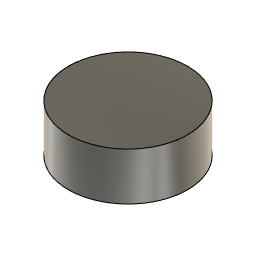
speed_meter (Autodesk Fusion 360 archive; units mm, degrees)
design "magnes"
Autodesk Fusion 360 part; units mm, degrees
note: some values were not read from the file. Chosen so that the rebuilt part matches the saved one: a direction; which face or edge a step refers to. Set by a fixed rule: which sketch regions a step uses.
sketch "Szkic1" plane through (0, 0, 0) normal (0, 0, 1) x (1, 0, 0)
  circle A0 centre (0, 0) radius 5
  dimension "d1" = 10
  constraint coincident A0.centre origin
  measures "d1" diameter of A0
extrude "Wyciągnięcie proste1" add sketch "Szkic1" along normal blind 4

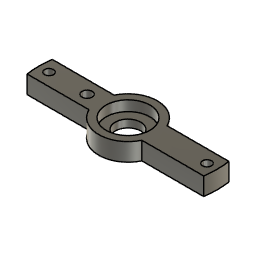
design "podstawa"
Autodesk Fusion 360 part; units mm, degrees
sketch "Szkic1" plane through (0, 0, 0) normal (0, 0, 1) x (1, 0, 0)
  circle A0 centre (0, 0) radius 11.5
  circle A1 centre (0, 0) radius 8.6
  circle A2 centre (0, 0) radius 5
  dimension "d1" = 23
  dimension "d2" = 17.2
  dimension "d7" = 10
  constraint coincident A0.centre A1.centre
  measures "d1" diameter of A0
  measures "d2" diameter of A1
  measures "d7" diameter of A2
extrude "Wyciągnięcie proste1" add sketch "Szkic1" along normal blind 7 contours A0
extrude "Wyciągnięcie proste2" add sketch "Szkic1" along normal blind 3 contours A1
sketch "Szkic2" plane through (0, 0, 0) normal (0, 0, 1) x (1, 0, 0)
  line L0 (20, -5) -> (-20, -5)
  line L1 (-20, 5) -> (20, 5)
  line L2 (20, -5) -> (-20, 5) construction
  line L3 (-20, -5) -> (20, 5) construction
  line L4 (35, -4.95) -> (-35, -4.95)
  line L5 (-35, -4.95) -> (-35, 4.95)
  line L6 (-35, 4.95) -> (35, 4.95)
  line L7 (35, 4.95) -> (35, -4.95)
  line L8 (35, -4.95) -> (-35, 4.95) construction
  line L9 (-20, -5) -> (-24, -5)
  line L10 (-24, 5) -> (-20, 5)
  circle A0 centre (0, 0) radius 11.5
  line L11 (-35, -4.95) -> (-11.3867, -1.6104) construction
  line L12 (0, 0) -> (35, 4.95) construction
  circle A1 centre (0, 0) radius 35
  circle A2 centre (-31, 0) radius 1.75
  circle A3 centre (31, 0) radius 1.75
  circle A4 centre (-15.9999, -0.05) radius 2
  dimension "d9" = 10
  dimension "d10" = 70
  dimension "d11" = 9.9
  dimension "d36" = 3.5
  dimension "d37" = 4
  dimension "d38" = 4
  dimension "d68" = 4
  dimension "d69" = 5
  dimension "d70" = 16
  constraint horizontal L0
  constraint parallel L0 L1
  constraint coincident L2 A0.centre
  constraint coincident L3 A0.centre
  constraint coincident A0.centre L12.start
  constraint horizontal L4
  constraint perpendicular L4 L5
  constraint parallel L4 L6
  constraint parallel L5 L7
  constraint coincident L8 A0.centre
  constraint coincident A0.centre L11
  constraint horizontal L9
  constraint horizontal L10
  constraint coincident A0 L11.end
  constraint collinear L11 L12
  constraint tangent L7 A1
  constraint horizontal A0.centre A3.centre
  constraint horizontal A0.centre A2.centre
  constraint equal A2 A3
  measures "d9" distance of L0.end L1.start
  measures "d10" distance of L5.end L6.end
  measures "d11" distance of L4.end L5.end
  measures "d36" diameter of A3
  measures "d37" distance of L7 A3.centre
  measures "d38" distance of L5 A2.centre
  measures "d68" diameter of A4
  measures "d69" distance of L6 A4.centre
  measures "d70" distance of A0.centre A4.centre
extrude "Wyciągnięcie proste3" add sketch "Szkic2" along normal blind 7 contours L4 L6 A0 A1 | L4 L6 A0 A1

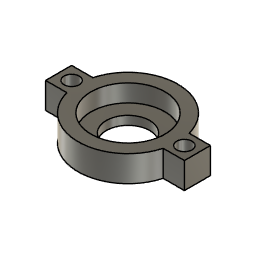
design "uchwyt lozysko"
Autodesk Fusion 360 part; units mm, degrees
sketch "Szkic1" plane through (0, 0, 0) normal (0, 0, 1) x (1, 0, 0)
  circle A0 centre (0, 0) radius 5
  circle A1 centre (0, 0) radius 8.5
  circle A2 centre (0, 0) radius 11.5
  circle A3 centre (13, 0) radius 1.75
  circle A4 centre (-13, 0) radius 1.75
  line L0 (16, 3) -> (-16, 3)
  line L1 (-16, 3) -> (-16, -3)
  line L2 (-16, -3) -> (16, -3)
  line L3 (16, -3) -> (16, 3)
  line L4 (16, 3) -> (-16, -3) construction
  line L5 (-16, 3) -> (16, -3) construction
  dimension "d1" = 10
  dimension "d2" = 17
  dimension "d3" = 23
  dimension "d4" = 3.5
  dimension "d5" = 13
  dimension "d6" = 3.5
  dimension "d7" = 13
  dimension "d8" = 32
  dimension "d9" = 6
  constraint coincident A0.centre A1.centre
  constraint concentric A0 A2
  constraint horizontal L0
  constraint perpendicular L0 L1
  constraint parallel L0 L2
  constraint parallel L1 L3
  constraint coincident L4 A0.centre
  constraint coincident L5 A0.centre
  constraint horizontal A0.centre A4.centre
  constraint horizontal A0.centre A3.centre
  measures "d1" diameter of A0
  measures "d2" diameter of A1
  measures "d3" diameter of A2
  measures "d4" diameter of A3
  measures "d5" distance of A0.centre A3.centre
  measures "d6" diameter of A4
  measures "d7" distance of A0.centre A4.centre
  measures "d8" distance of L1.end L2.end
  measures "d9" distance of L0.end L1.end
extrude "Wyciągnięcie proste1" add sketch "Szkic1" along normal blind 6 contours A1 A2 A3 L0 L2 | A1 A2 L0 | A1 A2 L2 | A1 A2 A4 L0 L2 | A2 A3 L0 L2 L3 | A2 A4 L0 L1 L2
extrude "Wyciągnięcie proste2" add sketch "Szkic1" along normal blind 2 contours A0 A1 L0 L2 | A0 A1 L0 | A0 A1 L2 | A0 A1 L0 L2

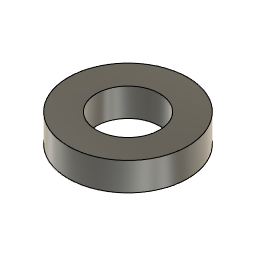
design "lozysko"
Autodesk Fusion 360 part; units mm, degrees
sketch "Szkic1" plane through (0, 0, 0) normal (0, 0, 1) x (1, 0, 0)
  circle A0 centre (0, 0) radius 4.5
  circle A1 centre (0, 0) radius 8.5
  dimension "d1" = 9
  dimension "d2" = 17
  constraint coincident A0.centre A1.centre
  constraint concentric A0 A1
  measures "d1" diameter of A0
  measures "d2" diameter of A1
extrude "Wyciągnięcie proste1" add sketch "Szkic1" along normal blind 4

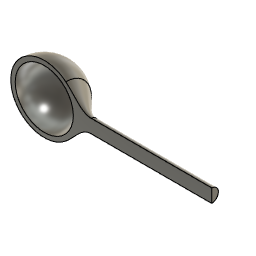
design "lopatka"
Autodesk Fusion 360 part; units mm, degrees
sketch "Szkic1" plane through (0, 0, 0) normal (0, 1, 0) x (1, 0, 0)
  line L0 (13, 0) -> (15, 0)
  line L1 (0, 0) -> (-15, 0)
  arc A0 (-15, 0) -> (15, 0) centre (0, 0) ccw
  arc A1 (-13, 0) -> (13, 0) centre (0, 0) ccw
  dimension "d1" = 30
  dimension "d2" = 26
  constraint coincident L1.start A0.centre
  constraint horizontal L0
  constraint parallel L0 L1
  constraint coincident L1 A1.start
  measures "d1" diameter of A0
  measures "d2" diameter of A1
revolve "Obrót1" add sketch "Szkic1" angle 180 about axis through (0, 0, 0) along (-1, 0, 0)
sketch "Szkic2" plane through (0, 0, 0) normal (0, 1, 0) x (1, 0, 0)
  line L0 (75, 0) -> (75, -3)
  line L1 (75, -3) -> (21, -3)
  spline S0 degree 5 poles (9.6157, -11.5125) (10.0753, -11.1286) (10.9799, -10.329) (12.293, -9.0341) (13.9792, -7.1799) (16.0934, -4.9797) (17.9027, -3.6587) (19.3902, -3.1198) (20.4518, -3) (21, -3) knots 0 0 0 0 0 0 0.2 0.4 0.6 0.8 1 1 1 1 1 1
  line L2 (8.6945, -12.2819) -> (10.5369, -10.7431)
  line L3 (20, -3) -> (22, -3)
  arc A0 (9.6157, -11.5125) -> (15, 0) centre (0, 0) ccw
  line L4 (15, 0) -> (75, 0)
  dimension "d9" = 60
  constraint vertical L0
  constraint horizontal L1
  constraint coincident A0.centre origin
  constraint midpoint S0.start L2
  constraint midpoint L1.end L3
  constraint coincident L1 L3.end
  constraint tangent L2 A0
  measures "d9" distance of A0.end L0.start
revolve "Obrót2" add sketch "Szkic2" angle 180 about axis through (1.75, 0, 0) along (-1, 0, 0) contours L0 L1 S0 L3 A0 L4

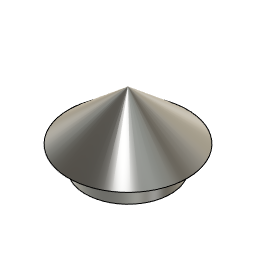
design "nakladka"
Autodesk Fusion 360 part; units mm, degrees
sketch "Szkic1" plane through (0, 0, 0) normal (0, 1, 0) x (1, 0, 0)
  line L0 (-6, 0) -> (0, -5.0346)
  line L1 (0, -3.3564) -> (0, -5.0346)
  line L2 (-2.5, 0) -> (1.3455, 0) construction
  line L3 (-2.5, 0) -> (0, -2.0977)
  line L4 (-2.5, 0) -> (1.1341, 0) construction
  line L5 (0, -2.0977) -> (0, -5.0346)
  line L6 (-2.5, 0) -> (-4, 1.2586)
  line L7 (-6, 0) -> (-4, 0) construction
  line L8 (-2.5, 0) -> (3.6054, 0) construction
  line L9 (-6, 0) -> (-8.0308, 1.704)
  line L10 (-8.0308, 1.704) -> (-6, 1.704)
  line L11 (-6, 1.704) -> (-5.75, 4.704)
  line L12 (-5.75, 4.704) -> (-4, 4.704)
  line L13 (-4, 4.704) -> (-4, 1.2586)
  dimension "d4" = 6
  dimension "d5" = 40
  dimension "d7" = 40
  dimension "d11" = 2
  dimension "d13" = 4
  dimension "d14" = 1.75
  dimension "d15" = 3
  constraint horizontal L7
  constraint perpendicular L1 L7
  constraint horizontal L2
  constraint coincident L2.start L7
  constraint horizontal L4
  constraint parallel L1 L5
  constraint parallel L3 L6
  constraint collinear L7 L8
  constraint parallel L0 L9
  constraint perpendicular L12 L13
  constraint vertical L13
  measures "d4" distance of origin L0.start
  measures "d5" angle of L0 L7
  measures "d7" angle of L3 L4
  measures "d11" horizontal distance of L6.end L10.end
  measures "d13" distance of origin L13
  measures "d14" distance of L11.end L12.end
  measures "d15" vertical distance of L10.end L11.end
revolve "Obrót1" add sketch "Szkic1" angle 360 about axis through (0, 0, 1.75) along (0, 0, 1)

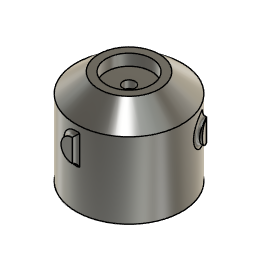
design "polaczenie predkosciomierz"
Autodesk Fusion 360 part; units mm, degrees
sketch "Szkic1" plane through (0, 0, 0) normal (0, 1, 0) x (1, 0, 0)
  line L0 (-14, -9.648) -> (-14, 10.352)
  line L1 (-14, -9.648) -> (-10.7329, -7.3965) construction
  line L2 (-14, -9.648) -> (-8, -14.6956)
  line L3 (-10, 10.352) -> (-10, -8.0131)
  line L4 (-10, -8.0131) -> (-8, -9.6956)
  line L5 (-14, 10.352) -> (-10, 10.352)
  line L6 (-10, 7.8472) -> (-14, 10.352) construction
  line L7 (0, -9.6956) -> (-8, -9.6956)
  line L8 (0, -14.6956) -> (-8, -14.6956)
  line L9 (0, -9.6956) -> (0, -14.6956)
  line L10 (0, 0) -> (0, -20.3833)
  line L11 (-4.9, -9.6956) -> (-4.9, -6.6956)
  line L12 (-4.9, -6.6956) -> (-10, -6.6956)
  dimension "d2" = 20
  dimension "d5" = 4
  dimension "d7" = 8
  dimension "d8" = 8
  dimension "d16" = 6
  dimension "d26" = 5
  dimension "d27" = 3
  dimension "d28" = 4.9
  constraint coincident L1 L10.start
  constraint coincident L10.start origin
  constraint perpendicular L3 L5
  constraint parallel L2 L4
  constraint coincident L3 L6.start
  constraint coincident L4 L1.end
  constraint horizontal L7
  constraint coincident L8.start L9.end
  constraint vertical L9
  constraint vertical L10
  constraint collinear L9 L10
  constraint coincident L7 L11.start
  constraint perpendicular L7 L11
  constraint coincident L3 L12.end
  constraint perpendicular L3 L12
  measures "d2" distance of L0.start L0.end
  measures "d5" distance of L0 L3
  measures "d7" distance of L7.start L4.end
  measures "d8" distance of L8.start L2.end
  measures "d16" horizontal distance of L0.start L4.end
  measures "d26" distance of L7 L8
  measures "d27" distance of L11.start L11.end
  measures "d28" horizontal distance of L10.start L11.end
revolve "Obrót1" add sketch "Szkic1" angle 360 about axis through (0, 0, 1.75) along (0, 0, 1)
sketch "Szkic2" plane through (0, 0, 14.6956) normal (0, 0, 1) x (-1, 0, 0)
  circle A0 centre (0, 0) radius 8
  circle A1 centre (0, 0) radius 1.6
  dimension "d9" = 3.2
  constraint coincident A0.centre A1.centre
  measures "d9" diameter of A1
extrude "Wyciągnięcie proste1" cut sketch "Szkic2" against normal blind 5.667 contours A1
sketch "Szkic3" plane through (0, 0, 14.6956) normal (0, 0, 1) x (-1, 0, 0)
  circle A0 centre (0, 0) radius 1.6
  circle A1 centre (0, 0) radius 8
  circle A2 centre (0, 0) radius 6
  dimension "d12" = 12
  constraint coincident A0.centre A1.centre
  measures "d12" diameter of A2
extrude "Wyciągnięcie proste2" cut sketch "Szkic3" against normal blind 3 contours A2
ref_plane "Płaszczyzna konstrukcyjna1" through (0, -14, -0.8921) normal (0, -1, 0) x (1, 0, 0)
sketch "Szkic4" plane through (0, -14, -0.8921) normal (0, -1, 0) x (1, 0, 0)
  line L0 (0, 8) -> (0, 2)
  arc A0 (0, 8) -> (0, 2) centre (0, 5) ccw
  constraint vertical L0
extrude "Wyciągnięcie proste3" add sketch "Szkic4" along normal blind 1 and the other way blind 1
fillet "Zaokrąglenie1" radius 1 2 edges at (-3, -13.6748, 4.1079) (0, -14, 4.1079)
pattern_circular "Szyk kołowy1" count 3 over 360 about axis through (0, 0, 1.75) along (0, 0, 1) of "Wyciągnięcie proste3", "Zaokrąglenie1"
